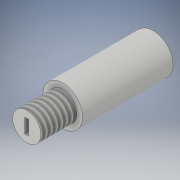
# Autodesk Inventor part: Pedal Shaft Extender Right
Saved by Autodesk Inventor 2019 (Build 230136000, 136)
## iProperties
Created: 2020-06-01
Part Number: Pedal Shaft Extender Right
Material: Generic
Document SubType Name: Modeling
Designer: 18186
Density: 1 g/cm^3
Appearance: Default
Author: 18186
Autodesk Inventor part; units mm, degrees
ref_plane "YZ Plane" through (0, 0, 0) normal (1, 0, 0) x (0, 1, 0)
ref_plane "XZ Plane" through (0, 0, 0) normal (0, 1, 0) x (-1, 0, 0)
ref_plane "XY Plane" through (0, 0, 0) normal (0, 0, 1) x (1, 0, 0)
sketch "Sketch1" plane through (0, 0, 0) normal (0, 0, 1) x (1, 0, 0)
  circle A0 centre (0, 0) radius 5
  circle A1 centre (0, 0) radius 7
  dimension "d0" = 10
  dimension "d1" = 14
  constraints: 2 centre point, 2 coincident
  measures "d0" diameter of A0
  measures "d1" diameter of A1
extrude "Extrusion1" add sketch "Sketch1" along normal blind 12.7
sketch "Sketch2" plane through (0, 0, 12.7) normal (0, 0, 1) x (1, 0, 0)
  circle A0 centre (0, 0) radius 7
  dimension "d14" = 14
  constraints: 1 centre point, 1 coincident
  measures "d14" diameter of A0
extrude "Extrusion2" add sketch "Sketch2" along normal blind 19.25
chamfer "Chamfer1" distance 0.4128 angle 45 1 edges at (-5, 0, 0)
thread "Thread1" size "7/16-14 UNC" class "2B" standard "ANSI Unified Screw Threads" full length
sketch "Sketch3" plane through (0, 0, 31.95) normal (0, 0, 1) x (1, 0, 0)
  circle A0 centre (0, 0) radius 5
  dimension "d11" = 10
  constraints: 1 centre point, 1 coincident
  measures "d11" diameter of A0
extrude "Extrusion3" add sketch "Sketch3" along normal blind 12.7
thread "Thread2" size "7/16-14 UNC" class "2A" standard "ANSI Unified Screw Threads" full length
sketch "Sketch4" plane through (0, 0, 44.65) normal (0, 0, 1) x (1, 0, 0)
  line L0 (0.635, -2.54) -> (-0.635, -2.54)
  line L1 (-0.635, -2.54) -> (-0.635, 2.54)
  line L2 (-0.635, 2.54) -> (0.635, 2.54)
  line L3 (0.635, 2.54) -> (0.635, -2.54)
  line L4 (0.635, -2.54) -> (-0.635, 2.54) construction
  line L5 (-0.635, -2.54) -> (0.635, 2.54) construction
  point P0 (0, 0)
  dimension "d17" = 1.27
  dimension "d18" = 5.08
  constraints: 12 end point, 2 midpoint, 2 parallel, 1 horizontal, 1 perpendicular
  measures "d17" distance of L1.end L2.end
  measures "d18" distance of L0.end L1.end
extrude "Extrusion4" cut sketch "Sketch4" against normal through all
body "Solid1"
